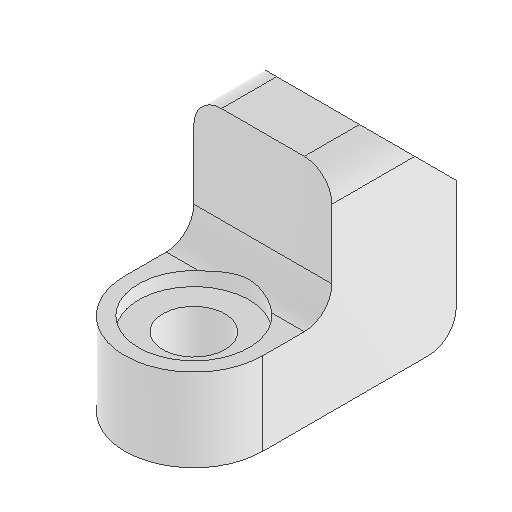
# Autodesk Inventor part: DLT-01-237
Saved by Autodesk Inventor 2025.2 (Build 292293000, 293)
## iProperties
Company: Delta
Created: 2025-01-27
Part Number: DLT-01-237
Material: Poliacetal WT
Document SubType Name: Modeling
Designer: Willian Pinheiro
Density: 1.4 g/cm^3
Appearance: Smooth - White
Description: Trava
Mass: 2.27217 g
Surface Area: 10.0558 cm^2
Volume: 1.62298 cm^3
Project: DLT-01
Dimensões: 10 x 15 x 19 mm
Total: 2
Author: Willian Pinheiro
Revision Number: 00
Autodesk Inventor part; units mm, degrees
ref_plane "YZ Plane" through (0, 0, 0) normal (1, 0, 0) x (0, 1, 0)
ref_plane "XZ Plane" through (0, 0, 0) normal (0, 1, 0) x (-1, 0, 0)
ref_plane "XY Plane" through (0, 0, 0) normal (0, 0, 1) x (1, 0, 0)
sketch "Sketch1" plane through (0, 0, 0) normal (0, 0, 1) x (1, 0, 0)
  circle A0 centre (0, 0) radius 5
  line L0 (-5, 0) -> (5, 0)
  line L1 (5, 0) -> (5, 14)
  line L2 (5, 14) -> (-5, 14)
  line L3 (-5, 14) -> (-5, 0)
  line L4 (-5, 5) -> (5, 5)
  circle A1 centre (0, 0) radius 2.25
  circle A2 centre (0, 0) radius 3.5
  point P0 (5, 0)
  dimension "d0" = 10
  dimension "d1" = 19
  dimension "d2" = 9
  dimension "d3" = 4.5
  dimension "d24" = 7
  constraints: 10 end point, 3 coincident, 2 centre point, 2 horizontal, 2 parallel, 2 point on line, 2 vertical, 1 perpendicular, 3 other
  measures "d2" distance between parallel lines of L2 L4
  measures "d3" diameter of A1
  measures "d24" diameter of A2
extrude "Extrusion1" add sketch "Sketch1" along normal blind 15
extrude "Extrusion2" cut sketch "Sketch1" against normal blind 9 from surface at 15 contours L0 A2 A0 | L3 L4 A0 | A0 L0 A2 | A0 L4 L1 | A2 L0 A1 | L0 A1 A2 | A1 L0 | L0 A1
sketch "Sketch2" plane through (0, 0, 6) normal (0, 0, 1) x (1, 0, 0)
  point P0 (0, 0)
hole "Hole1" at (0, 0, 6) direction (0, 0, -1) diameter 4.5 end through all counterbore diameter 8 counterbore depth 1 clearance for "Socket Head Cap Screw ISO 4762" size "M4" standard "ISO"
chamfer "Chamfer1" distance 5 angle 45 1 edges at (0, 14, 15)
fillet "Fillet1" radius 2 4 edges at (0, 5, 6) (0, 14, 0) (5, 7, 15) (-5, 7, 15)
body "Solid1"
